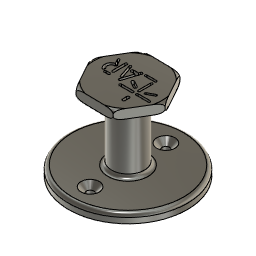
Suporte+Rolo+de+Estanho (Autodesk Fusion 360 design; units mm, degrees)
Autodesk Fusion 360 part; units mm, degrees
sketch "Esboço1" plane through (0, 0, 0) normal (0, 0, 1) x (1, 0, 0)
  circle A0 centre (0, 0) radius 9
  circle A1 centre (0, 0) radius 32.5
  circle A2 centre (0, 0) radius 20.75
  line L0 (10.0331, -18.1632) -> (20.7463, -0.3927)
  line L1 (20.7463, -0.3927) -> (10.7132, 17.7705)
  line L2 (10.7132, 17.7705) -> (-10.0331, 18.1632)
  line L3 (-10.0331, 18.1632) -> (-20.7463, 0.3927)
  line L4 (-20.7463, 0.3927) -> (-10.7132, -17.7705)
  line L5 (-10.7132, -17.7705) -> (10.0331, -18.1632)
  circle A3 centre (0, -20.75) radius 2
  circle A4 centre (0, 20.75) radius 2
  circle A5 centre (0, 0) radius 6
  dimension "d1" = 18
  dimension "d2" = 65
  dimension "d7" = 41.5
  dimension "d10" = 20.75
  dimension "d11" = 4
  dimension "d12" = 20.75
  dimension "d14" = 360
  dimension "d15" = 12
  constraint coincident A0.centre A1.centre
  constraint concentric A0 A1
  constraint concentric A1 A2
  constraint coincident A2 A3.centre
  measures "d1" diameter of A0
  measures "d2" diameter of A1
  measures "d7" diameter of A2
  measures "d10" distance of L0.start A0.centre
  measures "d11" diameter of A3
  measures "d12" vertical distance of A0.centre A3.centre
  measures "d15" diameter of A5
extrude "Extrusão1" add sketch "Esboço1" along normal blind 5 contours A1 | A2 L1 | A2 L2 A4 | L0 L1 L2 L3 L4 L5 | A2 L0 | A2 L3 | A2 L5 A3 | A2 L4 makes body 1
extrude "Extrusão2" add sketch "Esboço1" along normal blind 40 contours A0 | A5 bodies 1
extrude "Extrusão3" cut sketch "Esboço1" against normal blind 15 from surface at 40 contours A5 bodies 1
thread "Rosca1" "ISO Metric profile 12.0 M12x1.75 6H" major diameter 12.2265 minor diameter 10.2735 pitch 1.75 angle 60 modelled right hand crest width 0.4769 on face at (5.9702, -0.5974, 30) crest through (5.1368, 0, 39.5625) on bodies 1
extrude "Extrusão4" add sketch "Esboço1" along normal blind 5 from surface at 40 separate body contours A0 | A2 L1 | A2 L2 A4 | L0 L1 L2 L3 L4 L5 | A2 L0 | A2 A4 | A2 L3 | A2 L5 A3 | A2 L4 | A2 A3 | A5 picked at (-0.0483, 20.0779) picked at (-0.0483, -20.0779) makes body 2
fillet "Arredondamento1" radius 2 4 edges at (-30.3006, -11.7525, 5) (-8.3909, 3.2545, 5) (-19.3458, -7.5035, 45) (-19.3458, -7.5035, 40) on bodies 1 2
extrude "Extrusão5" cut sketch "Esboço1" along normal blind 5 from surface at 40 contours A0 | L0 L1 L2 L3 L4 L5 | A5 keep common part bodies 2
extrude "Extrusão6" add sketch "Esboço1" against normal blind 12 from surface at 40 contours A5 bodies 2
thread "Rosca2" "ISO Metric profile 12.0 M12x1.75 6g" major diameter 11.8335 minor diameter 9.8365 pitch 1.75 angle 60 modelled right hand crest width 0.2518 on face at (5.9925, -0.2991, 32) crest through (5.9168, 0, 40.4375) on bodies 2
chamfer "Chanfro1" distance 3 angle 45 2 edges at (-1.8647, -20.0268, 5) (-1.8647, 21.4732, 5) on bodies 1
sketch "Esboço2" plane through (0, 0, 45) normal (0, 0, 1) x (-1, 0, 0)
  line L0 (12.6266, -13.8612) -> (18.1527, -4.6947)
  arc A0 (18.1527, -4.6947) -> (18.3174, 4.0044) centre (0, 0) ccw
  line L1 (18.3174, 4.0044) -> (13.1421, 13.3734)
  arc A1 (13.1421, 13.3734) -> (5.6908, 17.8655) centre (0, 0) ccw
  line L2 (5.6908, 17.8655) -> (-5.0106, 18.0681)
  arc A2 (-5.0106, 18.0681) -> (-12.6266, 13.8612) centre (0, 0) ccw
  line L3 (-12.6266, 13.8612) -> (-18.1527, 4.6947)
  arc A3 (-18.1527, 4.6947) -> (-18.3174, -4.0044) centre (0, 0) ccw
  line L4 (-18.3174, -4.0044) -> (-13.1421, -13.3734)
  arc A4 (-13.1421, -13.3734) -> (-5.6908, -17.8655) centre (0, 0) ccw
  line L5 (-5.6908, -17.8655) -> (5.0106, -18.0681)
  arc A5 (5.0106, -18.0681) -> (12.6266, -13.8612) centre (0, 0) ccw
  line L6 (-7.9276, -7.271) -> (-2.5276, -7.271) construction
  arc A6 (3.4724, -6.4988) -> (3.4724, -4.9932) centre (3.4724, -5.746) ccw
  arc A7 (-0.7433, -6.899) -> (0.4882, -7.2985) centre (-0.1276, -7.0988) ccw
  line L7 (0.3113, -5.746) -> (3.4724, -5.746) construction
  line L8 (0.4882, -7.2985) -> (3.3473, 1.5156)
  line L9 (6.6574, -7.2864) -> (4.2877, -0.0833)
  line L10 (-8.6596, 10.3012) -> (-8.6596, 7.9012)
  line L11 (13.0235, -7.2923) -> (11.1307, -3.8879)
  line L12 (-5.5068, 0.4736) -> (-2.1783, -1.4821)
  line L13 (10.7113, -4.1212) -> (12.6041, -7.5255) construction
  arc A8 (4.2877, -0.0833) -> (3.2403, -0.4278) centre (3.764, -0.2555) ccw
  line L14 (2.1159, 1.9151) -> (-0.7433, -6.899)
  line L15 (7.7996, -0.3729) -> (7.7996, -7.4118)
  arc A9 (11.1307, -3.8879) -> (10.2918, -4.3544) centre (10.7113, -4.1212) ccw
  line L16 (-7.3575, -5.0889) -> (-7.3575, 1.9012)
  line L17 (0.3113, -6.4988) -> (3.4724, -6.4988)
  arc A10 (10.6579, -4.8323) -> (12.9434, 1.2613) centre (10.7018, -1.3733) ccw
  arc A11 (8.4566, 2.4579) -> (8.4566, 1.3012) centre (8.4566, 1.8796) ccw
  line L18 (-11.1866, 1.7837) -> (-14.9604, -0.2424)
  line L19 (-15.7276, 3.4985) -> (-9.0468, 3.4985)
  line L20 (0.1037, 4.6951) -> (-6.5832, 4.6951)
  arc A12 (9.1135, -0.3729) -> (7.7996, -0.3729) centre (8.4566, -0.3729) ccw
  line L21 (-6.5832, 4.0616) -> (0.1037, 4.0616) construction
  arc A13 (-9.0468, 3.4985) -> (-9.0468, 4.6717) centre (-9.0468, 4.0851) ccw
  arc A14 (-7.9276, -6.7079) -> (-7.9276, -7.8341) centre (-7.9276, -7.271) ccw
  arc A15 (-15.7276, 4.6717) -> (-15.7276, 3.4985) centre (-15.7276, 4.0851) ccw
  line L22 (-2.5276, -6.7079) -> (-7.9276, -6.7079)
  arc A16 (12.1846, -7.7587) -> (13.0235, -7.2923) centre (12.6041, -7.5255) ccw
  line L23 (-14.7014, -0.7248) -> (-10.9276, 1.3012) construction
  line L24 (-8.4976, 1.9012) -> (-8.4976, -5.0889)
  line L25 (-7.9276, 10.3012) -> (-7.9276, 7.9012) construction
  arc A17 (0.1037, 3.4281) -> (0.1037, 4.6951) centre (0.1037, 4.0616) ccw
  line L26 (8.4566, -0.3729) -> (8.4566, -7.4118) construction
  line L27 (10.2918, -4.3544) -> (12.1846, -7.7587)
  arc A18 (-8.6596, 7.9012) -> (-7.1955, 7.9012) centre (-7.9276, 7.9012) ccw
  line L28 (8.4566, 1.3012) -> (10.6724, 1.3012)
  line L29 (-1.4053, -0.1665) -> (-4.7339, 1.7891)
  arc A19 (-6.5832, 4.6951) -> (-6.5832, 3.4281) centre (-6.5832, 4.0616) ccw
  arc A20 (10.676, -3.4096) -> (10.6579, -4.8323) centre (10.667, -4.121) ccw
  line L30 (-5.1203, 1.1314) -> (-1.7918, -0.8243) construction
  line L31 (3.764, -0.2555) -> (6.1337, -7.4587) construction
  line L32 (8.4566, 1.8796) -> (10.6724, 1.8796) construction
  arc A21 (-7.3575, 1.9012) -> (-8.4976, 1.9012) centre (-7.9276, 1.9012) ccw
  arc A22 (-10.6686, 0.8188) -> (-11.1866, 1.7837) centre (-10.9276, 1.3012) ccw
  line L33 (3.4724, -4.9932) -> (0.3113, -4.9932)
  arc A23 (3.3473, 1.5156) -> (2.1159, 1.9151) centre (2.7316, 1.7153) ccw
  line L34 (-7.9276, 1.9012) -> (-7.9276, -5.0889) construction
  arc A24 (-2.1783, -1.4821) -> (-1.4053, -0.1665) centre (-1.7918, -0.8243) ccw
  arc A25 (0.3113, -4.9932) -> (0.3113, -6.4988) centre (0.3113, -5.746) ccw
  arc A26 (-7.1955, 10.3012) -> (-8.6596, 10.3012) centre (-7.9276, 10.3012) ccw
  arc A27 (5.61, -7.631) -> (6.6574, -7.2864) centre (6.1337, -7.4587) ccw
  line L35 (10.6724, 2.4579) -> (8.4566, 2.4579)
  line L36 (-0.1276, -7.0988) -> (2.7316, 1.7153) construction
  line L37 (-7.9276, -7.8341) -> (-2.5276, -7.8341)
  line L38 (3.2403, -0.4278) -> (5.61, -7.631)
  arc A28 (12.9434, 1.2613) -> (12.0214, 0.1776) centre (12.4824, 0.7195) ccw
  arc A29 (-2.5276, -7.8341) -> (-2.5276, -6.7079) centre (-2.5276, -7.271) ccw
  line L39 (-9.0468, 4.0851) -> (-15.7276, 4.0851) construction
  arc A30 (10.667, -4.121) -> (12.4824, 0.7195) centre (10.7018, -1.3733) ccw construction
  arc A31 (-4.7339, 1.7891) -> (-5.5068, 0.4736) centre (-5.1203, 1.1314) ccw
  arc A32 (7.7996, -7.4118) -> (9.1135, -7.4118) centre (8.4566, -7.4118) ccw
  line L40 (-9.0468, 4.6717) -> (-15.7276, 4.6717)
  line L41 (-7.1955, 7.9012) -> (-7.1955, 10.3012)
  arc A33 (10.6724, 1.3012) -> (10.6724, 2.4579) centre (10.6724, 1.8796) ccw
  line L42 (9.1135, -7.4118) -> (9.1135, -0.3729)
  arc A34 (-8.4976, -5.0889) -> (-7.3575, -5.0889) centre (-7.9276, -5.0889) ccw
  line L43 (-14.4424, -1.2072) -> (-10.6686, 0.8188)
  arc A35 (-14.9604, -0.2424) -> (-14.4424, -1.2072) centre (-14.7014, -0.7248) ccw
  arc A36 (10.676, -3.4096) -> (12.0214, 0.1776) centre (10.7018, -1.3733) ccw
  line L44 (-6.5832, 3.4281) -> (0.1037, 3.4281)
  point P0 (2.5, -10)
  point P1 (3.0547, -10.1032)
  constraint tangent L10 A18
  constraint tangent A18 L41
  constraint parallel L10 L41
  constraint tangent A26 L41
  constraint tangent L10 A26
  constraint tangent A17 L44
  constraint tangent L20 A17
  constraint parallel L20 L44
  constraint tangent L20 A19
  constraint tangent A19 L44
  constraint tangent L12 A24
  constraint tangent L29 A24
  constraint parallel L12 L29
  constraint tangent L29 A31
  constraint tangent L12 A31
  constraint tangent L24 A34
  constraint tangent L16 A34
  constraint parallel L16 L24
  constraint tangent L16 A21
  constraint tangent L24 A21
  constraint tangent A22 L43
  constraint tangent L18 A22
  constraint parallel L18 L43
  constraint tangent L18 A35
  constraint tangent L43 A35
  constraint tangent A15 L40
  constraint tangent L19 A15
  constraint parallel L19 L40
  constraint tangent L19 A13
  constraint tangent A13 L40
  constraint perpendicular L24 L39
  constraint tangent L37 A29
  constraint tangent L22 A29
  constraint parallel L22 L37
  constraint tangent A14 L22
  constraint tangent A14 L37
  constraint perpendicular L6 L24
  constraint tangent L8 A23
  constraint tangent L14 A23
  constraint parallel L8 L14
  constraint tangent A7 L14
  constraint tangent A7 L8
  constraint tangent A6 L17
  constraint tangent A6 L33
  constraint parallel L17 L33
  constraint tangent L33 A25
  constraint tangent L17 A25
  constraint coincident L7.start L36
  constraint tangent A27 L38
  constraint tangent L9 A27
  constraint parallel L9 L38
  constraint tangent L9 A8
  constraint tangent A8 L38
  constraint tangent L15 A32
  constraint tangent A32 L42
  constraint parallel L15 L42
  constraint tangent A12 L42
  constraint tangent L15 A12
  constraint tangent L28 A33
  constraint tangent L35 A33
  constraint parallel L28 L35
  constraint tangent A11 L35
  constraint tangent A11 L28
  constraint tangent A10 A20
  constraint tangent A20 A36
  constraint tangent A28 A36
  constraint tangent A10 A28
  constraint tangent A16 L27
  constraint tangent L11 A16
  constraint parallel L11 L27
  constraint tangent L11 A9
  constraint tangent A9 L27
  constraint coincident L13.start A30
extrude "Extrusão7" cut sketch "Esboço2" against normal blind 2 contours A6 L8 L17 L33 | L8 L14 L17 L33 A25 | A7 L8 L14 L17 A25 | L8 L14 L33 A23 A25 | L14 A25 | L9 A8 A27 L38 | L10 A18 A26 L41 | L11 A10 A16 L27 A20 | L11 A9 A10 L27 A20 | L11 A9 A10 L27 A20 A28 A36 | L12 L29 A24 A31 | L15 A12 A32 L42 | L16 L24 A21 A34 | A11 L28 L35 A33 | L18 A22 L43 A35 | L19 A13 A15 L40 | L20 A17 A19 L44 | A14 L22 L37 A29 bodies 2
equation "d3 = 5 mm"
equation "d5 = 35 mm + d3"
equation "d7 = ( d2 + d1 ) / 2"
equation "d10 = ( d2 + d1 ) / 4"
equation "d12 = ( d2 + d1 ) / 4"
equation "d16 = d5"
equation "d19 = d5"
equation "d22 = d5"
equation "d25 = d5"
named bodies: "Suporte", "Parafuso"
